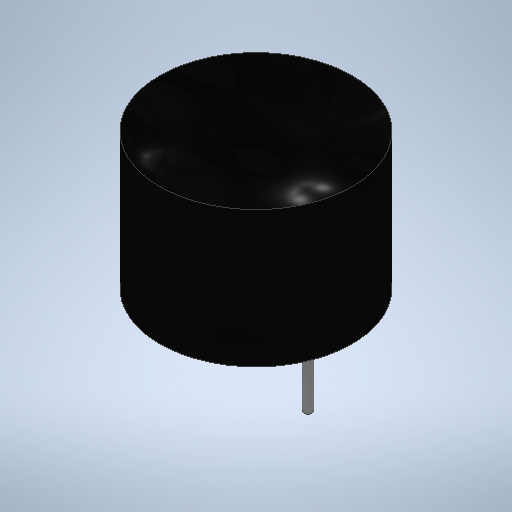
# Autodesk Inventor part: Buzzer
Saved by Autodesk Inventor 2025.2 (Build 292293000, 293)
## iProperties
Created: 2026-02-19
Part Number: Buzzer
Material: 一般
Document SubType Name: Modeling
Designer: naka6
Density: 1 g/cm^3
Appearance: 既定
Author: naka6
Autodesk Inventor part; units mm, degrees
ref_plane "YZ Plane" through (0, 0, 0) normal (1, 0, 0) x (0, 1, 0)
ref_plane "XZ Plane" through (0, 0, 0) normal (0, 1, 0) x (-1, 0, 0)
ref_plane "XY Plane" through (0, 0, 0) normal (0, 0, 1) x (1, 0, 0)
sketch "スケッチ1" plane through (0, 0, 0) normal (0, 1, 0) x (-1, 0, 0)
  circle A0 centre (0, 0) radius 6
  dimension "d0" = 12
  constraints: 1 centre point, 1 coincident
  measures "d0" diameter of A0
extrude "押し出し1" add sketch "スケッチ1" along normal blind 8.5
sketch "スケッチ2" plane through (0, 0, 0) normal (0, -1, 0) x (1, 0, 0)
  circle A0 centre (0, 0) radius 3.25
  line L0 (-5.9563, 0) -> (5.7903, 0)
  circle A1 centre (-3.25, 0) radius 0.25
  circle A2 centre (3.25, 0) radius 0.25
  dimension "d3" = 6.5
  dimension "d4" = 0.5
  dimension "d5" = 0.5
  constraints: 3 centre point, 3 coincident, 2 end point, 2 point on circle, 2 point on line, 1 horizontal
  measures "d3" diameter of A0
  measures "d4" diameter of A1
  measures "d5" diameter of A2
extrude "押し出し2" add sketch "スケッチ2" along normal blind 5 contours L0 A2 A0 | L0 A2 A0 | A0 A2 L0 | A0 A2 L0 | A1 L0 A0 | A0 L0 A1 | A1 L0 A0 | A0 L0 A1
